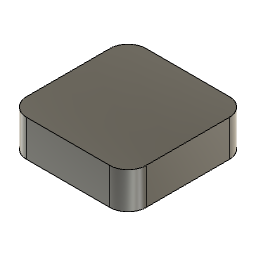
MiniPi (Autodesk Fusion 360 archive; units mm, degrees)
design "USB Power Supply"
Autodesk Fusion 360 part; units mm, degrees
sketch "Sketch1" plane through (0, 0, 0) normal (0, 0, 1) x (1, 0, 0) in component "Component"
  line L0 (82, 82) -> (-82, 82)
  line L1 (-82, 82) -> (-82, -82)
  line L2 (-82, -82) -> (82, -82)
  line L3 (82, -82) -> (82, 82)
  line L4 (82, 82) -> (-82, -82) construction
  line L5 (-82, 82) -> (82, -82) construction
  dimension "d1" = 164
  dimension "d2" = 164
  constraint horizontal L0
  constraint perpendicular L0 L1
  constraint parallel L0 L2
  constraint parallel L1 L3
  constraint coincident L4 origin
  constraint coincident L5 origin
  measures "d1" distance of L1.end L2.end
  measures "d2" distance of L0.end L1.end
extrude "Extrude1" add sketch "Sketch1" along normal blind 50 in component "Component"
fillet "Fillet1" radius 25 4 edges at (82, -82, 25) (-82, 82, 25) (-82, -82, 25) (82, 82, 25) in component "Component"
component "Component" placed x (1, 0, 0) y (0, 1, 0) z (0, 0, 1) at (0, 0, 0)

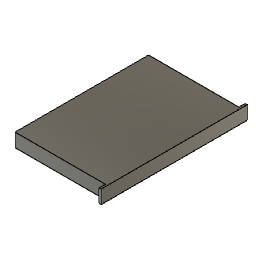
design "Switch"
Autodesk Fusion 360 part; units mm, degrees
sketch "Sketch1" plane through (0, 0, 0) normal (0, 0, 1) x (1, 0, 0)
  line L0 (152.4, 241.3) -> (-152.4, 241.3)
  line L1 (-152.4, 241.3) -> (-152.4, -241.3)
  line L2 (-152.4, -241.3) -> (152.4, -241.3)
  line L3 (152.4, -241.3) -> (152.4, 241.3)
  line L4 (152.4, 241.3) -> (-152.4, -241.3) construction
  line L5 (-152.4, 241.3) -> (152.4, -241.3) construction
  dimension "d1" = 304.8
  dimension "d2" = 482.6
  constraint perpendicular L0 L1
  constraint parallel L0 L2
  constraint parallel L1 L3
  constraint horizontal L0
  constraint coincident L4 origin
  constraint coincident L5 origin
  measures "d1" distance of L1.end L2.end
  measures "d2" distance of L0.end L1.end
extrude "Extrude1" add sketch "Sketch1" along normal blind 44.45
sketch "Sketch2" plane through (0, 0, 44.45) normal (0, 0, 1) x (-1, 0, 0)
  line L0 (-152.4, 241.3) -> (-152.4, -241.3)
  line L1 (-152.4, -241.3) -> (152.4, -241.3)
  line L2 (152.4, -241.3) -> (152.4, 241.3)
  line L3 (152.4, 241.3) -> (-152.4, 241.3)
  line L4 (-145.6, -241.3) -> (152.4, -241.3)
  line L5 (152.4, -241.3) -> (152.4, -220.3)
  line L6 (152.4, -220.3) -> (-145.6, -220.3)
  line L7 (-145.6, -220.3) -> (-145.6, -241.3)
  line L8 (-145.6, 241.3) -> (152.4, 241.3)
  line L9 (152.4, 241.3) -> (152.4, 220.3)
  line L10 (152.4, 220.3) -> (-145.6, 220.3)
  line L11 (-145.6, 220.3) -> (-145.6, 241.3)
  dimension "d5" = 21
  dimension "d6" = 21
  dimension "d7" = 298
  dimension "d8" = 298
  dimension "d11" = 6.8
  dimension "d12" = 6.8
  constraint horizontal L4
  constraint vertical L5
  constraint horizontal L6
  constraint vertical L7
  constraint coincident L1 L4.start
  constraint horizontal L8
  constraint vertical L9
  constraint horizontal L10
  constraint vertical L11
  constraint coincident L3 L8.start
  measures "d5" distance of L4.start L6.end
  measures "d6" distance of L8.start L10.end
  measures "d7" distance of L8.start L2.end
  measures "d8" distance of L5 L7
  measures "d11" distance of L0 L11
  measures "d12" distance of L0 L7
extrude "Extrude2" cut sketch "Sketch2" against normal up to surface (44.45 mm away) contours L2 L3 L8 L9 L10 L11 | L1 L2 L4 L5 L6 L7
equation "d11 = 1 ft - 298 mm"
equation "d12 = 1 ft - 298 mm"

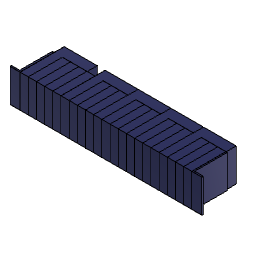
design "2UPi with Fans"
Autodesk Fusion 360 part; units mm, degrees
sketch "Sketch1" plane through (-215.9, 0, 0) normal (1, 0, 0) x (0, 1, 0) in component "1"
  line L0 (-42.8625, 0) -> (42.8625, 0)
  line L1 (42.8625, 0) -> (42.8625, 83)
  line L2 (42.8625, 83) -> (-42.8625, 83)
  line L3 (-42.8625, 83) -> (-42.8625, 0)
  line L4 (-42.8625, 83) -> (42.8625, 83)
  line L5 (42.8625, 83) -> (42.8625, 0)
  line L6 (42.8625, 0) -> (-42.8625, 0)
  line L7 (-42.8625, 0) -> (-42.8625, 83)
  constraint horizontal L4
  constraint vertical L5
  constraint horizontal L6
  constraint vertical L7
  constraint coincident L0.end L1.start
  constraint coincident L2.end L3.start
extrude "Extrude1" add sketch "Sketch1" along normal blind 20.57 makes body 1 in component "1"
sketch "Sketch1 (2)" plane through (-195.33, 0, 0) normal (1, 0, 0) x (0, 1, 0) in component "2"
  line L0 (-42.8625, 0) -> (42.8625, 0)
  line L1 (42.8625, 0) -> (42.8625, 83)
  line L2 (42.8625, 83) -> (-42.8625, 83)
  line L3 (-42.8625, 83) -> (-42.8625, 0)
  line L4 (-42.8625, 83) -> (42.8625, 83)
  line L5 (42.8625, 83) -> (42.8625, 0)
  line L6 (42.8625, 0) -> (-42.8625, 0)
  line L7 (-42.8625, 0) -> (-42.8625, 83)
  constraint horizontal L4
  constraint vertical L5
  constraint horizontal L6
  constraint vertical L7
  constraint coincident L0.end L1.start
  constraint coincident L2.end L3.start
extrude "Extrude1'" add sketch "Sketch1 (2)" along normal blind 20.57 separate body makes body 2 in component "2"
sketch "Sketch1 (3)" plane through (-174.76, 0, 0) normal (1, 0, 0) x (0, 1, 0) in component "3"
  line L0 (-42.8625, 0) -> (42.8625, 0)
  line L1 (42.8625, 0) -> (42.8625, 83)
  line L2 (42.8625, 83) -> (-42.8625, 83)
  line L3 (-42.8625, 83) -> (-42.8625, 0)
  line L4 (-42.8625, 83) -> (42.8625, 83)
  line L5 (42.8625, 83) -> (42.8625, 0)
  line L6 (42.8625, 0) -> (-42.8625, 0)
  line L7 (-42.8625, 0) -> (-42.8625, 83)
  constraint horizontal L4
  constraint vertical L5
  constraint horizontal L6
  constraint vertical L7
  constraint coincident L0.end L1.start
  constraint coincident L2.end L3.start
extrude "Extrude1''" add sketch "Sketch1 (3)" along normal blind 20.57 separate body makes body 3 in component "3"
sketch "Sketch1 (4)" plane through (-154.19, 0, 0) normal (1, 0, 0) x (0, 1, 0) in component "4"
  line L0 (-42.8625, 0) -> (42.8625, 0)
  line L1 (42.8625, 0) -> (42.8625, 83)
  line L2 (42.8625, 83) -> (-42.8625, 83)
  line L3 (-42.8625, 83) -> (-42.8625, 0)
  line L4 (-42.8625, 83) -> (42.8625, 83)
  line L5 (42.8625, 83) -> (42.8625, 0)
  line L6 (42.8625, 0) -> (-42.8625, 0)
  line L7 (-42.8625, 0) -> (-42.8625, 83)
  constraint horizontal L4
  constraint vertical L5
  constraint horizontal L6
  constraint vertical L7
  constraint coincident L0.end L1.start
  constraint coincident L2.end L3.start
extrude "Extrude1'''" add sketch "Sketch1 (4)" along normal blind 20.57 separate body makes body 4 in component "4"
sketch "Sketch1 (5)" plane through (-133.62, 0, 0) normal (1, 0, 0) x (0, 1, 0) in component "5"
  line L0 (-42.8625, 0) -> (42.8625, 0)
  line L1 (42.8625, 0) -> (42.8625, 83)
  line L2 (42.8625, 83) -> (-42.8625, 83)
  line L3 (-42.8625, 83) -> (-42.8625, 0)
  line L4 (-42.8625, 83) -> (42.8625, 83)
  line L5 (42.8625, 83) -> (42.8625, 0)
  line L6 (42.8625, 0) -> (-42.8625, 0)
  line L7 (-42.8625, 0) -> (-42.8625, 83)
  constraint horizontal L4
  constraint vertical L5
  constraint horizontal L6
  constraint vertical L7
  constraint coincident L0.end L1.start
  constraint coincident L2.end L3.start
extrude "Extrude1''''" add sketch "Sketch1 (5)" along normal blind 20.57 separate body makes body 5 in component "5"
sketch "Sketch1 (6)" plane through (-113.05, 0, 0) normal (1, 0, 0) x (0, 1, 0) in component "6"
  line L0 (-42.8625, 0) -> (42.8625, 0)
  line L1 (42.8625, 0) -> (42.8625, 83)
  line L2 (42.8625, 83) -> (-42.8625, 83)
  line L3 (-42.8625, 83) -> (-42.8625, 0)
  line L4 (-42.8625, 83) -> (42.8625, 83)
  line L5 (42.8625, 83) -> (42.8625, 0)
  line L6 (42.8625, 0) -> (-42.8625, 0)
  line L7 (-42.8625, 0) -> (-42.8625, 83)
  constraint horizontal L4
  constraint vertical L5
  constraint horizontal L6
  constraint vertical L7
  constraint coincident L0.end L1.start
  constraint coincident L2.end L3.start
extrude "Extrude1'''''" add sketch "Sketch1 (6)" along normal blind 20.57 separate body makes body 6 in component "6"
sketch "Sketch1 (7)" plane through (-92.48, 0, 0) normal (1, 0, 0) x (0, 1, 0) in component "7"
  line L0 (-42.8625, 0) -> (42.8625, 0)
  line L1 (42.8625, 0) -> (42.8625, 83)
  line L2 (42.8625, 83) -> (-42.8625, 83)
  line L3 (-42.8625, 83) -> (-42.8625, 0)
  line L4 (-42.8625, 83) -> (42.8625, 83)
  line L5 (42.8625, 83) -> (42.8625, 0)
  line L6 (42.8625, 0) -> (-42.8625, 0)
  line L7 (-42.8625, 0) -> (-42.8625, 83)
  constraint horizontal L4
  constraint vertical L5
  constraint horizontal L6
  constraint vertical L7
  constraint coincident L0.end L1.start
  constraint coincident L2.end L3.start
extrude "Extrude1''''''" add sketch "Sketch1 (7)" along normal blind 20.57 separate body makes body 7 in component "7"
sketch "Sketch1 (8)" plane through (-71.91, 0, 0) normal (1, 0, 0) x (0, 1, 0) in component "8"
  line L0 (-42.8625, 0) -> (42.8625, 0)
  line L1 (42.8625, 0) -> (42.8625, 83)
  line L2 (42.8625, 83) -> (-42.8625, 83)
  line L3 (-42.8625, 83) -> (-42.8625, 0)
  line L4 (-42.8625, 83) -> (42.8625, 83)
  line L5 (42.8625, 83) -> (42.8625, 0)
  line L6 (42.8625, 0) -> (-42.8625, 0)
  line L7 (-42.8625, 0) -> (-42.8625, 83)
  constraint horizontal L4
  constraint vertical L5
  constraint horizontal L6
  constraint vertical L7
  constraint coincident L0.end L1.start
  constraint coincident L2.end L3.start
extrude "Extrude1'''''''" add sketch "Sketch1 (8)" along normal blind 20.57 separate body makes body 8 in component "8"
sketch "Sketch1 (9)" plane through (-51.34, 0, 0) normal (1, 0, 0) x (0, 1, 0) in component "9"
  line L0 (-42.8625, 0) -> (42.8625, 0)
  line L1 (42.8625, 0) -> (42.8625, 83)
  line L2 (42.8625, 83) -> (-42.8625, 83)
  line L3 (-42.8625, 83) -> (-42.8625, 0)
  line L4 (-42.8625, 83) -> (42.8625, 83)
  line L5 (42.8625, 83) -> (42.8625, 0)
  line L6 (42.8625, 0) -> (-42.8625, 0)
  line L7 (-42.8625, 0) -> (-42.8625, 83)
  constraint horizontal L4
  constraint vertical L5
  constraint horizontal L6
  constraint vertical L7
  constraint coincident L0.end L1.start
  constraint coincident L2.end L3.start
extrude "Extrude1''''''''" add sketch "Sketch1 (9)" along normal blind 20.57 separate body makes body 9 in component "9"
sketch "Sketch1 (10)" plane through (-30.77, 0, 0) normal (1, 0, 0) x (0, 1, 0) in component "10"
  line L0 (-42.8625, 0) -> (42.8625, 0)
  line L1 (42.8625, 0) -> (42.8625, 83)
  line L2 (42.8625, 83) -> (-42.8625, 83)
  line L3 (-42.8625, 83) -> (-42.8625, 0)
  line L4 (-42.8625, 83) -> (42.8625, 83)
  line L5 (42.8625, 83) -> (42.8625, 0)
  line L6 (42.8625, 0) -> (-42.8625, 0)
  line L7 (-42.8625, 0) -> (-42.8625, 83)
  constraint horizontal L4
  constraint vertical L5
  constraint horizontal L6
  constraint vertical L7
  constraint coincident L0.end L1.start
  constraint coincident L2.end L3.start
extrude "Extrude1'''''''''" add sketch "Sketch1 (10)" along normal blind 20.57 separate body makes body 10 in component "10"
sketch "Sketch1 (11)" plane through (-10.2, 0, 0) normal (1, 0, 0) x (0, 1, 0) in component "11"
  line L0 (-42.8625, 0) -> (42.8625, 0)
  line L1 (42.8625, 0) -> (42.8625, 83)
  line L2 (42.8625, 83) -> (-42.8625, 83)
  line L3 (-42.8625, 83) -> (-42.8625, 0)
  line L4 (-42.8625, 83) -> (42.8625, 83)
  line L5 (42.8625, 83) -> (42.8625, 0)
  line L6 (42.8625, 0) -> (-42.8625, 0)
  line L7 (-42.8625, 0) -> (-42.8625, 83)
  constraint horizontal L4
  constraint vertical L5
  constraint horizontal L6
  constraint vertical L7
  constraint coincident L0.end L1.start
  constraint coincident L2.end L3.start
extrude "Extrude1''''''''''" add sketch "Sketch1 (11)" along normal blind 20.57 separate body makes body 11 in component "11"
sketch "Sketch1 (12)" plane through (10.37, 0, 0) normal (1, 0, 0) x (0, 1, 0) in component "12"
  line L0 (-42.8625, 0) -> (42.8625, 0)
  line L1 (42.8625, 0) -> (42.8625, 83)
  line L2 (42.8625, 83) -> (-42.8625, 83)
  line L3 (-42.8625, 83) -> (-42.8625, 0)
  line L4 (-42.8625, 83) -> (42.8625, 83)
  line L5 (42.8625, 83) -> (42.8625, 0)
  line L6 (42.8625, 0) -> (-42.8625, 0)
  line L7 (-42.8625, 0) -> (-42.8625, 83)
  constraint horizontal L4
  constraint vertical L5
  constraint horizontal L6
  constraint vertical L7
  constraint coincident L0.end L1.start
  constraint coincident L2.end L3.start
extrude "Extrude1'''''''''''" add sketch "Sketch1 (12)" along normal blind 20.57 separate body makes body 12 in component "12"
sketch "Sketch1 (13)" plane through (30.94, 0, 0) normal (1, 0, 0) x (0, 1, 0) in component "13"
  line L0 (-42.8625, 0) -> (42.8625, 0)
  line L1 (42.8625, 0) -> (42.8625, 83)
  line L2 (42.8625, 83) -> (-42.8625, 83)
  line L3 (-42.8625, 83) -> (-42.8625, 0)
  line L4 (-42.8625, 83) -> (42.8625, 83)
  line L5 (42.8625, 83) -> (42.8625, 0)
  line L6 (42.8625, 0) -> (-42.8625, 0)
  line L7 (-42.8625, 0) -> (-42.8625, 83)
  constraint horizontal L4
  constraint vertical L5
  constraint horizontal L6
  constraint vertical L7
  constraint coincident L0.end L1.start
  constraint coincident L2.end L3.start
extrude "Extrude1''''''''''''" add sketch "Sketch1 (13)" along normal blind 20.57 separate body makes body 13 in component "13"
sketch "Sketch1 (14)" plane through (51.51, 0, 0) normal (1, 0, 0) x (0, 1, 0) in component "14"
  line L0 (-42.8625, 0) -> (42.8625, 0)
  line L1 (42.8625, 0) -> (42.8625, 83)
  line L2 (42.8625, 83) -> (-42.8625, 83)
  line L3 (-42.8625, 83) -> (-42.8625, 0)
  line L4 (-42.8625, 83) -> (42.8625, 83)
  line L5 (42.8625, 83) -> (42.8625, 0)
  line L6 (42.8625, 0) -> (-42.8625, 0)
  line L7 (-42.8625, 0) -> (-42.8625, 83)
  constraint horizontal L4
  constraint vertical L5
  constraint horizontal L6
  constraint vertical L7
  constraint coincident L0.end L1.start
  constraint coincident L2.end L3.start
extrude "Extrude1'''''''''''''" add sketch "Sketch1 (14)" along normal blind 20.57 separate body makes body 14 in component "14"
sketch "Sketch1 (15)" plane through (72.08, 0, 0) normal (1, 0, 0) x (0, 1, 0) in component "15"
  line L0 (-42.8625, 0) -> (42.8625, 0)
  line L1 (42.8625, 0) -> (42.8625, 83)
  line L2 (42.8625, 83) -> (-42.8625, 83)
  line L3 (-42.8625, 83) -> (-42.8625, 0)
  line L4 (-42.8625, 83) -> (42.8625, 83)
  line L5 (42.8625, 83) -> (42.8625, 0)
  line L6 (42.8625, 0) -> (-42.8625, 0)
  line L7 (-42.8625, 0) -> (-42.8625, 83)
  constraint horizontal L4
  constraint vertical L5
  constraint horizontal L6
  constraint vertical L7
  constraint coincident L0.end L1.start
  constraint coincident L2.end L3.start
extrude "Extrude1''''''''''''''" add sketch "Sketch1 (15)" along normal blind 20.57 separate body makes body 15 in component "15"
sketch "Sketch1 (16)" plane through (92.65, 0, 0) normal (1, 0, 0) x (0, 1, 0) in component "16"
  line L0 (-42.8625, 0) -> (42.8625, 0)
  line L1 (42.8625, 0) -> (42.8625, 83)
  line L2 (42.8625, 83) -> (-42.8625, 83)
  line L3 (-42.8625, 83) -> (-42.8625, 0)
  line L4 (-42.8625, 83) -> (42.8625, 83)
  line L5 (42.8625, 83) -> (42.8625, 0)
  line L6 (42.8625, 0) -> (-42.8625, 0)
  line L7 (-42.8625, 0) -> (-42.8625, 83)
  constraint horizontal L4
  constraint vertical L5
  constraint horizontal L6
  constraint vertical L7
  constraint coincident L0.end L1.start
  constraint coincident L2.end L3.start
extrude "Extrude1'''''''''''''''" add sketch "Sketch1 (16)" along normal blind 20.57 separate body makes body 16 in component "16"
sketch "Sketch1 (17)" plane through (113.22, 0, 0) normal (1, 0, 0) x (0, 1, 0) in component "17"
  line L0 (-42.8625, 0) -> (42.8625, 0)
  line L1 (42.8625, 0) -> (42.8625, 83)
  line L2 (42.8625, 83) -> (-42.8625, 83)
  line L3 (-42.8625, 83) -> (-42.8625, 0)
  line L4 (-42.8625, 83) -> (42.8625, 83)
  line L5 (42.8625, 83) -> (42.8625, 0)
  line L6 (42.8625, 0) -> (-42.8625, 0)
  line L7 (-42.8625, 0) -> (-42.8625, 83)
  constraint horizontal L4
  constraint vertical L5
  constraint horizontal L6
  constraint vertical L7
  constraint coincident L0.end L1.start
  constraint coincident L2.end L3.start
extrude "Extrude1''''''''''''''''" add sketch "Sketch1 (17)" along normal blind 20.57 separate body makes body 17 in component "17"
sketch "Sketch1 (18)" plane through (133.79, 0, 0) normal (1, 0, 0) x (0, 1, 0) in component "18"
  line L0 (-42.8625, 0) -> (42.8625, 0)
  line L1 (42.8625, 0) -> (42.8625, 83)
  line L2 (42.8625, 83) -> (-42.8625, 83)
  line L3 (-42.8625, 83) -> (-42.8625, 0)
  line L4 (-42.8625, 83) -> (42.8625, 83)
  line L5 (42.8625, 83) -> (42.8625, 0)
  line L6 (42.8625, 0) -> (-42.8625, 0)
  line L7 (-42.8625, 0) -> (-42.8625, 83)
  constraint horizontal L4
  constraint vertical L5
  constraint horizontal L6
  constraint vertical L7
  constraint coincident L0.end L1.start
  constraint coincident L2.end L3.start
extrude "Extrude1'''''''''''''''''" add sketch "Sketch1 (18)" along normal blind 20.57 separate body makes body 18 in component "18"
sketch "Sketch1 (19)" plane through (154.36, 0, 0) normal (1, 0, 0) x (0, 1, 0) in component "19"
  line L0 (-42.8625, 0) -> (42.8625, 0)
  line L1 (42.8625, 0) -> (42.8625, 83)
  line L2 (42.8625, 83) -> (-42.8625, 83)
  line L3 (-42.8625, 83) -> (-42.8625, 0)
  line L4 (-42.8625, 83) -> (42.8625, 83)
  line L5 (42.8625, 83) -> (42.8625, 0)
  line L6 (42.8625, 0) -> (-42.8625, 0)
  line L7 (-42.8625, 0) -> (-42.8625, 83)
  constraint horizontal L4
  constraint vertical L5
  constraint horizontal L6
  constraint vertical L7
  constraint coincident L0.end L1.start
  constraint coincident L2.end L3.start
extrude "Extrude1''''''''''''''''''" add sketch "Sketch1 (19)" along normal blind 20.57 separate body makes body 19 in component "19"
sketch "Sketch1 (20)" plane through (174.93, 0, 0) normal (1, 0, 0) x (0, 1, 0) in component "20"
  line L0 (-42.8625, 0) -> (42.8625, 0)
  line L1 (42.8625, 0) -> (42.8625, 83)
  line L2 (42.8625, 83) -> (-42.8625, 83)
  line L3 (-42.8625, 83) -> (-42.8625, 0)
  line L4 (-42.8625, 83) -> (42.8625, 83)
  line L5 (42.8625, 83) -> (42.8625, 0)
  line L6 (42.8625, 0) -> (-42.8625, 0)
  line L7 (-42.8625, 0) -> (-42.8625, 83)
  constraint horizontal L4
  constraint vertical L5
  constraint horizontal L6
  constraint vertical L7
  constraint coincident L0.end L1.start
  constraint coincident L2.end L3.start
extrude "Extrude1'''''''''''''''''''" add sketch "Sketch1 (20)" along normal blind 20.57 separate body makes body 20 in component "20"
sketch "Sketch1 (21)" plane through (195.5, 0, 0) normal (1, 0, 0) x (0, 1, 0) in component "21"
  line L0 (-42.8625, 0) -> (42.8625, 0)
  line L1 (42.8625, 0) -> (42.8625, 83)
  line L2 (42.8625, 83) -> (-42.8625, 83)
  line L3 (-42.8625, 83) -> (-42.8625, 0)
  line L4 (-42.8625, 83) -> (42.8625, 83)
  line L5 (42.8625, 83) -> (42.8625, 0)
  line L6 (42.8625, 0) -> (-42.8625, 0)
  line L7 (-42.8625, 0) -> (-42.8625, 83)
  constraint horizontal L4
  constraint vertical L5
  constraint horizontal L6
  constraint vertical L7
  constraint coincident L0.end L1.start
  constraint coincident L2.end L3.start
extrude "Extrude1''''''''''''''''''''" add sketch "Sketch1 (21)" along normal blind 20.57 separate body makes body 21 in component "21"
sketch "Sketch1 (22)" plane through (0, 0, 0) normal (0, 0, 1) x (1, 0, 0) in component "Component'''''''''"
  line L0 (-241.3, -42.8625) -> (241.3, -42.8625)
  line L1 (241.3, -42.8625) -> (241.3, 42.8625)
  line L2 (241.3, 42.8625) -> (-241.3, 42.8625)
  line L3 (-241.3, 42.8625) -> (-241.3, -42.8625)
  line L4 (-241.3, -42.8625) -> (241.3, 42.8625) construction
  line L5 (241.3, -42.8625) -> (-241.3, 42.8625) construction
  line L6 (-241.3, 42.8625) -> (-220.6671, 42.8625)
  line L7 (-220.6671, 42.8625) -> (-220.6671, -39.1974)
  line L8 (-220.6671, -39.1974) -> (-241.3, -39.1974)
  line L9 (-241.3, -39.1974) -> (-241.3, 42.8625)
  line L10 (-241.3, 42.8625) -> (-216.3, 42.8625)
  line L11 (-216.3, 42.8625) -> (-216.3, -42.8625)
  line L12 (-216.3, -42.8625) -> (-241.3, -42.8625)
  line L13 (-241.3, -42.8625) -> (-241.3, 42.8625)
  line L14 (241.3, 42.8625) -> (216.3, 42.8625)
  line L15 (216.3, 42.8625) -> (216.3, -42.8625)
  line L16 (216.3, -42.8625) -> (241.3, -42.8625)
  line L17 (241.3, -42.8625) -> (241.3, 42.8625)
  line L18 (241.3, 42.8625) -> (219.6466, 42.8625)
  line L19 (219.6466, 42.8625) -> (219.6466, -39.0162)
  line L20 (219.6466, -39.0162) -> (241.3, -39.0162)
  line L21 (241.3, -39.0162) -> (241.3, 42.8625)
  dimension "d50" = 482.6
  dimension "d51" = 85.725
  dimension "d52" = 25
  dimension "d53" = 25
  constraint perpendicular L0 L1
  constraint parallel L0 L2
  constraint parallel L1 L3
  constraint horizontal L0
  constraint coincident L4 origin
  constraint coincident L5 origin
  constraint horizontal L6
  constraint vertical L7
  constraint horizontal L8
  constraint vertical L9
  constraint coincident L4 L7.end
  constraint horizontal L10
  constraint vertical L11
  constraint horizontal L12
  constraint vertical L13
  constraint vertical L15
  constraint horizontal L16
  constraint vertical L19
  constraint horizontal L20
  constraint coincident L5 L19.end
  measures "d50" distance of L1.end L2.end
  measures "d51" distance of L0.end L1.end
  measures "d52" distance of L2.end L10.end
  measures "d53" distance of L1.end L14.end
extrude "Extrude1'''''''''''''''''''''" add sketch "Sketch1 (22)" along normal blind 83 separate body contours L0 L2 L3 L7 L8 L10 L11 L12 L13 | L0 L1 L2 L14 L15 L16 L17 L19 L20 makes body 22 at (216.3, 14.2875, 55.3333) makes body 23 at (-216.3, 14.2875, 55.3333) in component "Component'''''''''"
sketch "Sketch2" plane through (0, 42.8625, 0) normal (0, 1, 0) x (-1, 0, 0) in component "1"
  line L0 (215.9, 0) -> (215.9, 83)
  line L1 (215.9, 83) -> (195.33, 83)
  line L2 (195.33, 83) -> (195.33, 0)
  line L3 (195.33, 0) -> (215.9, 0)
  line L4 (215.9, 83) -> (132.9, 83)
  line L5 (132.9, 83) -> (132.9, 0)
  line L6 (132.9, 0) -> (215.9, 0)
  line L7 (215.9, 0) -> (215.9, 83)
  circle A0 centre (174.4, 41.5) radius 35
  dimension "d56" = 83
  dimension "d57" = 70
  dimension "d58" = 41.5
  dimension "d59" = 41.5
  constraint horizontal L4
  constraint vertical L5
  constraint horizontal L6
  constraint vertical L7
  constraint coincident L0.end L1.start
  measures "d56" distance of L0.end L4.end
  measures "d57" diameter of A0
  measures "d58" distance of L6 A0.centre
  measures "d59" distance of L5 A0.centre
extrude "Extrude2" add sketch "Sketch2" along normal blind 25.4 contours L0 L1 L2 L3 L4 L6 L7 A0 | L2 L4 L5 L6 A0 bodies 1 in component "1"
sketch "Sketch2 (2)" plane through (0, 42.8625, 0) normal (0, 1, 0) x (-1, 0, 0) in component "6"
  line L0 (113.05, 0) -> (113.05, 83)
  line L1 (113.05, 83) -> (92.48, 83)
  line L2 (92.48, 83) -> (92.48, 0)
  line L3 (92.48, 0) -> (113.05, 0)
  line L4 (113.05, 83) -> (30.05, 83)
  line L5 (30.05, 83) -> (30.05, 0)
  line L6 (30.05, 0) -> (113.05, 0)
  line L7 (113.05, 0) -> (113.05, 83)
  circle A0 centre (71.55, 41.5) radius 35
  dimension "d62" = 83
  dimension "d63" = 70
  dimension "d64" = 41.5
  dimension "d65" = 41.5
  constraint horizontal L4
  constraint vertical L5
  constraint horizontal L6
  constraint vertical L7
  constraint coincident L0.end L1.start
  measures "d62" distance of L0.end L4.end
  measures "d63" diameter of A0
  measures "d64" distance of L6 A0.centre
  measures "d65" distance of L7 A0.centre
extrude "Extrude2'" add sketch "Sketch2 (2)" along normal blind 25.4 contours L0 L1 L2 L3 L4 L6 L7 A0 | L2 L4 L5 L6 A0 bodies 6 in component "6"
sketch "Sketch2 (3)" plane through (0, 42.8625, 0) normal (0, 1, 0) x (-1, 0, 0) in component "10"
  line L0 (30.77, 0) -> (30.77, 83)
  line L1 (30.77, 83) -> (10.2, 83)
  line L2 (10.2, 83) -> (10.2, 0)
  line L3 (10.2, 0) -> (30.77, 0)
  line L4 (30.77, 83) -> (-52.23, 83)
  line L5 (-52.23, 83) -> (-52.23, 0)
  line L6 (-52.23, 0) -> (30.77, 0)
  line L7 (30.77, 0) -> (30.77, 83)
  circle A0 centre (-11.45, 41.5) radius 35
  line L8 (30.05, 83) -> (30.05, 0)
  dimension "d68" = 83
  dimension "d69" = 70
  dimension "d70" = 41.5
  dimension "d71" = 41.5
  constraint horizontal L4
  constraint vertical L5
  constraint horizontal L6
  constraint vertical L7
  constraint coincident L0.end L1.start
  measures "d68" distance of L0.end L4.end
  measures "d69" diameter of A0
  measures "d70" distance of A0.centre L8
  measures "d71" distance of L6 A0.centre
extrude "Extrude2''" add sketch "Sketch2 (3)" along normal blind 25.4 contours L1 L2 L3 L4 L6 A0 L8 | L2 L4 L5 L6 A0 bodies 10 in component "10"
sketch "Sketch2 (4)" plane through (0, 42.8625, 0) normal (0, 1, 0) x (-1, 0, 0) in component "14"
  line L0 (-51.51, 0) -> (-51.51, 83)
  line L1 (-51.51, 83) -> (-72.08, 83)
  line L2 (-72.08, 83) -> (-72.08, 0)
  line L3 (-72.08, 0) -> (-51.51, 0)
  line L4 (-51.51, 83) -> (-134.51, 83)
  line L5 (-134.51, 83) -> (-134.51, 0)
  line L6 (-134.51, 0) -> (-51.51, 0)
  line L7 (-51.51, 0) -> (-51.51, 83)
  circle A0 centre (-93.73, 41.5) radius 35
  line L8 (-52.23, 83) -> (-52.23, 0)
  dimension "d74" = 83
  dimension "d75" = 70
  dimension "d76" = 41.5
  dimension "d77" = 41.5
  constraint horizontal L4
  constraint vertical L5
  constraint horizontal L6
  constraint vertical L7
  constraint coincident L0.end L1.start
  measures "d74" distance of L0.end L4.end
  measures "d75" diameter of A0
  measures "d76" distance of L6 A0.centre
  measures "d77" distance of A0.centre L8
extrude "Extrude2'''" add sketch "Sketch2 (4)" along normal blind 25.4 contours L1 L2 L3 L4 L6 A0 L8 | L2 L4 L5 L6 A0 bodies 14 in component "14"
sketch "Sketch2 (5)" plane through (0, 42.8625, 0) normal (0, 1, 0) x (-1, 0, 0) in component "18"
  line L0 (-133.79, 0) -> (-133.79, 83)
  line L1 (-133.79, 83) -> (-154.36, 83)
  line L2 (-154.36, 83) -> (-154.36, 0)
  line L3 (-154.36, 0) -> (-133.79, 0)
  line L4 (-133.79, 83) -> (-216.79, 83)
  line L5 (-216.79, 83) -> (-216.79, 0)
  line L6 (-216.79, 0) -> (-133.79, 0)
  line L7 (-133.79, 0) -> (-133.79, 83)
  circle A0 centre (-176.01, 41.5) radius 35
  line L8 (-134.51, 83) -> (-134.51, 0)
  dimension "d80" = 83
  dimension "d81" = 70
  dimension "d82" = 41.5
  dimension "d83" = 41.5
  constraint horizontal L4
  constraint vertical L5
  constraint horizontal L6
  constraint vertical L7
  constraint coincident L0.end L1.start
  measures "d80" distance of L0.end L4.end
  measures "d81" diameter of A0
  measures "d82" distance of L6 A0.centre
  measures "d83" distance of A0.centre L8
extrude "Extrude2''''" add sketch "Sketch2 (5)" along normal blind 25.4 contours L1 L2 L3 L4 L6 A0 L8 | L2 L4 L5 L6 A0 bodies 18 in component "18"
component "1" placed x (1, 0, 0) y (0, 1, 0) z (0, 0, 1) at (0, 0, 0)
component "2" placed x (1, 0, 0) y (0, 1, 0) z (0, 0, 1) at (0, 0, 0)
component "3" placed x (1, 0, 0) y (0, 1, 0) z (0, 0, 1) at (0, 0, 0)
component "4" placed x (1, 0, 0) y (0, 1, 0) z (0, 0, 1) at (0, 0, 0)
component "5" placed x (1, 0, 0) y (0, 1, 0) z (0, 0, 1) at (0, 0, 0)
component "6" placed x (1, 0, 0) y (0, 1, 0) z (0, 0, 1) at (0, 0, 0)
component "7" placed x (1, 0, 0) y (0, 1, 0) z (0, 0, 1) at (0, 0, 0)
component "8" placed x (1, 0, 0) y (0, 1, 0) z (0, 0, 1) at (0, 0, 0)
component "9" placed x (1, 0, 0) y (0, 1, 0) z (0, 0, 1) at (0, 0, 0)
component "10" placed x (1, 0, 0) y (0, 1, 0) z (0, 0, 1) at (0, 0, 0)
component "11" placed x (1, 0, 0) y (0, 1, 0) z (0, 0, 1) at (0, 0, 0)
component "12" placed x (1, 0, 0) y (0, 1, 0) z (0, 0, 1) at (0, 0, 0)
component "13" placed x (1, 0, 0) y (0, 1, 0) z (0, 0, 1) at (0, 0, 0)
component "14" placed x (1, 0, 0) y (0, 1, 0) z (0, 0, 1) at (0, 0, 0)
component "15" placed x (1, 0, 0) y (0, 1, 0) z (0, 0, 1) at (0, 0, 0)
component "16" placed x (1, 0, 0) y (0, 1, 0) z (0, 0, 1) at (0, 0, 0)
component "17" placed x (1, 0, 0) y (0, 1, 0) z (0, 0, 1) at (0, 0, 0)
component "18" placed x (1, 0, 0) y (0, 1, 0) z (0, 0, 1) at (0, 0, 0)
component "19" placed x (1, 0, 0) y (0, 1, 0) z (0, 0, 1) at (0, 0, 0)
component "20" placed x (1, 0, 0) y (0, 1, 0) z (0, 0, 1) at (0, 0, 0)
component "21" placed x (1, 0, 0) y (0, 1, 0) z (0, 0, 1) at (0, 0, 0)
component "Component'''''''''" placed x (1, 0, 0) y (0, 1, 0) z (0, 0, 1) at (0, 0, 0)
equation "d7 = w"
equation "d9 = w"
equation "d11 = w"
equation "d13 = w"
equation "d15 = w"
equation "d17 = w"
equation "d19 = w"
equation "w = 20.57 mm"
equation "d22 = w"
equation "d24 = w"
equation "d26 = w"
equation "d28 = w"
equation "d30 = w"
equation "d32 = w"
equation "d34 = w"
equation "d36 = w"
equation "d38 = w"
equation "d40 = w"
equation "d42 = w"
equation "d44 = w"
equation "d46 = w"
equation "d48 = w"
equation "d58 = ( 83 / 2 ) * 1 mm"
equation "d59 = ( 83 / 2 ) * 1 mm"
equation "d64 = ( 83 / 2 ) * 1 mm"
equation "d65 = ( 83 / 2 ) * 1 mm"
equation "d70 = ( 83 / 2 ) * 1 mm"
equation "d71 = ( 83 / 2 ) * 1 mm"
equation "d76 = ( 83 / 2 ) * 1 mm"
equation "d77 = ( 83 / 2 ) * 1 mm"
equation "d82 = ( 83 / 2 ) * 1 mm"
equation "d83 = ( 83 / 2 ) * 1 mm"

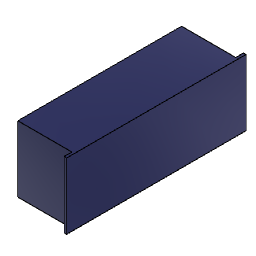
design "Mini Pi Server"
Autodesk Fusion 360 part; units mm, degrees
sketch "Sketch1" plane through (0, 0, 0) normal (0, 0, 1) x (1, 0, 0)
  line L0 (76.2, 241.3) -> (-76.2, 241.3)
  line L1 (-76.2, 241.3) -> (-76.2, -241.3)
  line L2 (-76.2, -241.3) -> (76.2, -241.3)
  line L3 (76.2, -241.3) -> (76.2, 241.3)
  line L4 (76.2, 241.3) -> (-76.2, -241.3) construction
  line L5 (-76.2, 241.3) -> (76.2, -241.3) construction
  dimension "d1" = 152.4
  dimension "d2" = 482.6
  constraint perpendicular L0 L1
  constraint parallel L0 L2
  constraint parallel L1 L3
  constraint horizontal L0
  constraint coincident L4 origin
  constraint coincident L5 origin
  measures "d1" distance of L1.end L2.end
  measures "d2" distance of L0.end L1.end
extrude "Extrude1" add sketch "Sketch1" along normal blind 177.8
sketch "Sketch2" plane through (0, 0, 177.8) normal (0, 0, 1) x (-1, 0, 0)
  line L0 (-76.2, 241.3) -> (-76.2, -241.3)
  line L1 (-76.2, -241.3) -> (76.2, -241.3)
  line L2 (76.2, -241.3) -> (76.2, 241.3)
  line L3 (76.2, 241.3) -> (-76.2, 241.3)
  line L4 (-69.4, -241.3) -> (228.6, -241.3)
  line L5 (228.6, -241.3) -> (228.6, -220.3)
  line L6 (228.6, -220.3) -> (-69.4, -220.3)
  line L7 (-69.4, -220.3) -> (-69.4, -241.3)
  line L8 (-69.4, 241.3) -> (228.6, 241.3)
  line L9 (228.6, 241.3) -> (228.6, 220.3)
  line L10 (228.6, 220.3) -> (-69.4, 220.3)
  line L11 (-69.4, 220.3) -> (-69.4, 241.3)
  dimension "d5" = 21
  dimension "d6" = 21
  dimension "d7" = 298
  dimension "d8" = 298
  dimension "d11" = 6.8
  dimension "d12" = 6.8
  constraint horizontal L4
  constraint vertical L5
  constraint horizontal L6
  constraint vertical L7
  constraint coincident L1 L4.start
  constraint horizontal L8
  constraint vertical L9
  constraint horizontal L10
  constraint vertical L11
  constraint coincident L3 L8.start
  measures "d5" distance of L4.start L6.end
  measures "d6" distance of L8.start L10.end
  measures "d7" distance of L8.start L8.end
  measures "d8" distance of L5 L7
  measures "d11" distance of L0 L11
  measures "d12" distance of L0 L7
extrude "Extrude2" cut sketch "Sketch2" against normal up to surface (177.8 mm away) contours L2 L3 L8 L10 L11 | L1 L2 L4 L6 L7 | L2 L8 L9 L10 | L2 L4 L5 L6
equation "d11 = 1 ft - 298 mm"
equation "d12 = 1 ft - 298 mm"
